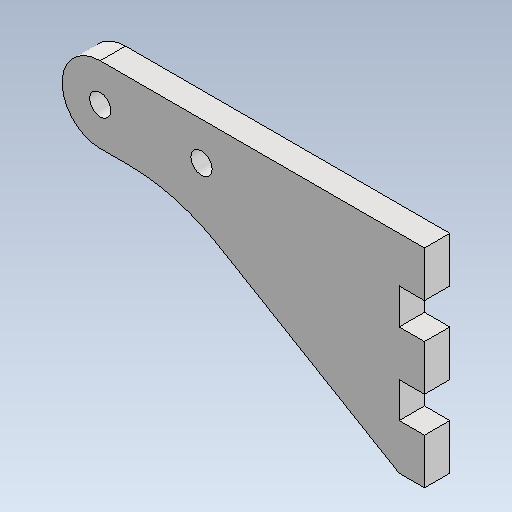
# Autodesk Inventor part: gate-upper-link
Saved by Autodesk Inventor 2025 (Build 290162000, 162)
## iProperties
Created: 2025-08-22
Part Number: gate-upper-link
Material: Generic
Document SubType Name: Modeling
Designer: HP
Density: 1 g/cm^3
Appearance: Default
Author: HP
Autodesk Inventor part; units mm, degrees
ref_plane "YZ Plane" through (0, 0, 0) normal (1, 0, 0) x (0, 1, 0)
ref_plane "XZ Plane" through (0, 0, 0) normal (0, 1, 0) x (-1, 0, 0)
ref_plane "XY Plane" through (0, 0, 0) normal (0, 0, 1) x (1, 0, 0)
sketch "Sketch1" plane through (0, 0, 0) normal (0, 0, 1) x (1, 0, 0)
  line L0 (-20, -7.5) -> (-5, -7.5)
  line L1 (44, 7.5) -> (-20, 7.5)
  arc A0 (-20, 7.5) -> (-20, -7.5) centre (-20, 0) ccw
  circle A1 centre (-20, 0) radius 2.1
  line L2 (44, 7.5) -> (44, -1.5)
  line L3 (39, -1.5) -> (39, -8.5)
  line L4 (39, -8.5) -> (44, -8.5)
  line L5 (44, -8.5) -> (44, -17.5)
  line L6 (44, -17.5) -> (39, -17.5)
  line L7 (39, -1.5) -> (44, -1.5)
  circle A2 centre (0, 0) radius 2.1
  line L8 (39, -17.5) -> (39, -24.5)
  line L9 (39, -24.5) -> (44, -24.5)
  line L10 (44, -24.5) -> (44, -33.5)
  line L11 (44, -33.5) -> (39, -33.5)
  line L12 (39, -33.5) -> (-5, -7.5)
  dimension "d1" = 4.2
  dimension "d8" = 15
  dimension "d9" = 5
  dimension "d10" = 7
  dimension "d11" = 9
  dimension "d12" = 9
  dimension "d14" = 4.2
  dimension "d15" = 20
  dimension "d16" = 64
  dimension "d17" = 15
  dimension "d18" = 7
  dimension "d19" = 9
  constraints: 26 end point, 6 perpendicular, 3 centre point, 3 coincident, 3 vertical, 2 collinear, 2 parallel, 2 point on circle, 2 point on line, 2 tangent, 1 horizontal alignment
  measures "d1" diameter of A1
  measures "d8" distance between parallel lines of L0 L1
  measures "d9" distance between parallel lines of L2 L3
  measures "d10" distance between parallel lines of L4 L7
  measures "d11" distance between parallel lines of L7 L1
  measures "d12" distance between parallel lines of L6 L4
  measures "d14" diameter of A2
  measures "d15" distance of A2.centre A0.centre
  measures "d16" distance from line of L2 A0.centre
  measures "d17" horizontal distance of L0.end A0.centre
  measures "d18" distance between parallel lines of L9 L6
  measures "d19" distance between parallel lines of L11 L9
extrude "Extrusion1" add sketch "Sketch1" along normal blind 5
fillet "Fillet1" radius 35 1 edges at (-5, -7.5, 2.5)
equation "\"d1\" = d14"
equation "\"d12\" = d11"
equation "\"d18\" = d10"
equation "\"d19\" = d12"
body "Solid1"
